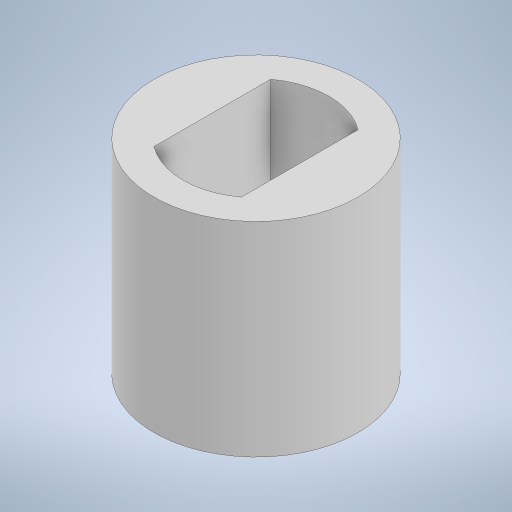
# Autodesk Inventor part: ozubeneKoleckoStepper
Saved by Autodesk Inventor 2023 (Build 270158000, 158)
## iProperties
Created: 2023-11-08
Part Number: ozubeneKoleckoStepper
Material: Generic
Document SubType Name: Modeling
Designer: alexa
Density: 1 g/cm^3
Appearance: Default
Author: alexa
Autodesk Inventor part; units mm, degrees
ref_plane "YZ Plane" through (0, 0, 0) normal (1, 0, 0) x (0, 1, 0)
ref_plane "XZ Plane" through (0, 0, 0) normal (0, 1, 0) x (-1, 0, 0)
ref_plane "XY Plane" through (0, 0, 0) normal (0, 0, 1) x (1, 0, 0)
sketch "Sketch1" plane through (0, 0, 0) normal (0, 1, 0) x (-1, 0, 0)
  circle A0 centre (0, 0) radius 3.5
  dimension "d0" = 7
  constraints: 1 centre point, 1 coincident
  measures "d0" diameter of A0
extrude "Extrusion1" add sketch "Sketch1" along normal blind 7
sketch "Sketch2" plane through (0, 7, 0) normal (0, 1, 0) x (1, 0, 0)
  circle A0 centre (0, 0) radius 2.5
  line L0 (1.5, -2.75) -> (-1.5, -2.75)
  line L1 (-1.5, -2.75) -> (-1.5, 2.75)
  line L2 (-1.5, 2.75) -> (1.5, 2.75)
  line L3 (1.5, 2.75) -> (1.5, -2.75)
  line L4 (1.5, -2.75) -> (-1.5, 2.75) construction
  line L5 (-1.5, -2.75) -> (1.5, 2.75) construction
  point P0 (1.5, -2)
  point P1 (1.5, 2)
  point P2 (-1.5, 2)
  point P3 (-1.5, -2)
  dimension "d3" = 5
  dimension "d4" = 3
  dimension "d5" = 5.5
  constraints: 12 end point, 2 midpoint, 2 parallel, 1 centre point, 1 coincident, 1 horizontal, 1 perpendicular
  measures "d3" diameter of A0
  measures "d4" distance of L1.end L2.end
  measures "d5" distance of L0.end L1.end
extrude "Extrusion2" cut sketch "Sketch2" against normal blind 6 contours L3 A0 L1
body "Solid1"
